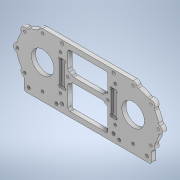
# Autodesk Inventor part: Trunk_lower_waisit_frame
Saved by Autodesk Inventor 2020.4 (Build 244396000, 396)
## iProperties
Created: 2021-09-21
Part Number: Trunk_lower_waisit_frame
Material: アルミニウム 2014-T4
Document SubType Name: Modeling
Designer: Masato Kubotera
Density: 2.8 g/cm^3
Appearance: 滑らか - 淡い灰色
Mass: 76.4309 g
Surface Area: 174.27 cm^2
Volume: 27.2967 cm^3
Description: A2017 T4
Author: Masato Kubotera
Autodesk Inventor part; units mm, degrees
ref_plane "YZ Plane" through (0, 0, 0) normal (1, 0, 0) x (0, 1, 0)
ref_plane "XZ Plane" through (0, 0, 0) normal (0, 1, 0) x (-1, 0, 0)
ref_plane "XY Plane" through (0, 0, 0) normal (0, 0, 1) x (1, 0, 0)
sketch "スケッチ1" plane through (0, 0, 0) normal (0, 0, 1) x (1, 0, 0)
  line L0 (-62, 30.75) -> (62, 30.75)
  line L1 (62, -30.75) -> (-62, -30.75)
  line L2 (-62, 30.75) -> (62, -30.75) construction
  line L3 (62, 30.75) -> (-62, -30.75) construction
  line L4 (0, 30.75) -> (0, -30.75) construction
  circle A0 centre (-44, 2.25) radius 10.5 construction
  line L5 (-57.5, 1.25) -> (-30.5, 1.25) construction
  line L6 (-30.5, 1.25) -> (-30.5, -25.75) construction
  line L7 (-30.5, -25.75) -> (-57.5, -25.75) construction
  line L8 (-57.5, -25.75) -> (-57.5, 1.25) construction
  line L9 (-44, 1.25) -> (-44, -25.75) construction
  line L10 (-57.5, -12.25) -> (-30.5, -12.25) construction
  circle A1 centre (-57.5, 1.25) radius 1.425 construction
  circle A2 centre (-57.5, -25.75) radius 1.425
  circle A3 centre (-30.5, 1.25) radius 1.425 construction
  circle A4 centre (-30.5, -25.75) radius 1.425
  line L11 (-27.5, 14.75) -> (-22.5, 14.75) construction
  line L12 (-22.5, 14.75) -> (-22.5, -10.25) construction
  line L13 (-22.5, -10.25) -> (-27.5, -10.25) construction
  line L14 (-27.5, -10.25) -> (-27.5, 14.75) construction
  line L15 (-27.5, 14.75) -> (-22.5, -10.25) construction
  line L16 (-22.5, 14.75) -> (-27.5, -10.25) construction
  line L17 (-27.51, 14.76) -> (-22.49, 14.76)
  line L18 (-22.49, 14.76) -> (-22.49, -10.26)
  line L19 (-22.49, -10.26) -> (-27.51, -10.26)
  line L20 (-27.51, -10.26) -> (-27.51, 14.76)
  line L21 (-27.51, 14.76) -> (-22.49, -10.26) construction
  line L22 (-22.49, 14.76) -> (-27.51, -10.26) construction
  line L23 (-27.51, 2.25) -> (-22.49, 2.25) construction
  line L24 (-25, 14.76) -> (-25, -10.26) construction
  arc A5 (-27.51, 14.76) -> (-27.51, 12.66) centre (-27.51, 13.71) ccw
  arc A6 (-22.49, 12.66) -> (-22.49, 14.76) centre (-22.49, 13.71) ccw
  arc A7 (-27.51, -8.16) -> (-27.51, -10.26) centre (-27.51, -9.21) ccw
  arc A8 (-22.49, -10.26) -> (-22.49, -8.16) centre (-22.49, -9.21) ccw
  circle A9 centre (-25, 27.75) radius 1.55
  line L25 (-22.5, -17.25) -> (-27.5, -17.25) construction
  circle A10 centre (-25, -23.25) radius 1.55
  circle A11 centre (-44, 2.25) radius 11
  line L26 (62, 2.25) -> (-62, 2.25) construction
  line L27 (-60, 14.25) -> (-28, 14.25) construction
  line L28 (-28, 14.25) -> (-28, -28.75) construction
  line L29 (-28, -28.75) -> (-60, -28.75) construction
  line L30 (-60, -28.75) -> (-60, 14.25) construction
  line L31 (-60, 14.25) -> (-28, -28.75) construction
  line L32 (-28, 14.25) -> (-60, -28.75) construction
  line L33 (-62, 30.75) -> (-62, -30.75) construction
  line L34 (62, 30.75) -> (62, -30.75) construction
  circle A12 centre (-44, 2.25) radius 12.5 construction
  circle A13 centre (-44, 2.25) radius 20.5 construction
  circle A14 centre (-44, 2.25) radius 28.5 construction
  circle A15 centre (-44, 26.75) radius 1.25
  circle A16 centre (-61.3241, 19.5741) radius 1.25
  circle A17 centre (-68.5, 2.25) radius 1.25
  circle A18 centre (-61.3241, -15.0741) radius 1.25
  circle A19 centre (-44, -22.25) radius 1.25
  circle A20 centre (-26.6759, -15.0741) radius 1.25
  circle A21 centre (-19.5, 2.25) radius 1.25
  circle A22 centre (-26.6759, 19.5741) radius 1.25
  line L35 (-62, -21.122) -> (-62, -30.75)
  circle A23 centre (57.5, 1.25) radius 1.425 construction
  circle A24 centre (57.5, -25.75) radius 1.425
  circle A25 centre (30.5, 1.25) radius 1.425 construction
  circle A26 centre (30.5, -25.75) radius 1.425
  line L36 (27.51, 14.76) -> (22.49, 14.76)
  line L37 (22.49, 14.76) -> (22.49, -10.26)
  line L38 (22.49, -10.26) -> (27.51, -10.26)
  line L39 (27.51, -10.26) -> (27.51, 14.76)
  arc A27 (27.51, 12.66) -> (27.51, 14.76) centre (27.51, 13.71) ccw
  arc A28 (22.49, 14.76) -> (22.49, 12.66) centre (22.49, 13.71) ccw
  arc A29 (22.49, -8.16) -> (22.49, -10.26) centre (22.49, -9.21) ccw
  arc A30 (27.51, -10.26) -> (27.51, -8.16) centre (27.51, -9.21) ccw
  circle A31 centre (25, 27.75) radius 1.55
  circle A32 centre (25, -23.25) radius 1.55
  circle A33 centre (44, 2.25) radius 11
  circle A34 centre (44, 26.75) radius 1.25
  circle A35 centre (61.3241, 19.5741) radius 1.25
  circle A36 centre (68.5, 2.25) radius 1.25
  circle A37 centre (61.3241, -15.0741) radius 1.25
  circle A38 centre (44, -22.25) radius 1.25
  circle A39 centre (26.6759, -15.0741) radius 1.25
  circle A40 centre (19.5, 2.25) radius 1.25
  circle A41 centre (26.6759, 19.5741) radius 1.25
  line L40 (62, -21.122) -> (62, -30.75)
  line L41 (-68.5, 2.25) -> (-73.5, 2.25) construction
  circle A42 centre (-26.6759, -15.0741) radius 6.25 construction
  circle A43 centre (-44, 2.25) radius 24.5 construction
  circle A44 centre (-30.5, -25.75) radius 2.4 construction
  arc A45 (-47.969, 27.2469) -> (-58.8689, 22.732) centre (-44, 2.25) ccw
  arc A46 (-44, 30.75) -> (-47.969, 27.2469) centre (-44, 26.75) ccw
  arc A47 (-58.8689, 22.732) -> (-64.482, 17.1189) centre (-61.3241, 19.5741) ccw
  arc A48 (-64.482, 17.1189) -> (-68.9969, 6.219) centre (-44, 2.25) ccw
  arc A49 (-68.9969, 6.219) -> (-68.9969, -1.719) centre (-68.5, 2.25) ccw
  arc A50 (-68.9969, -1.719) -> (-64.482, -12.6189) centre (-44, 2.25) ccw
  arc A51 (-64.482, -12.6189) -> (-62, -19.0166) centre (-61.3241, -15.0741) ccw
  line L42 (-62, -19.0166) -> (-62, -21.122)
  arc A52 (58.8689, 22.732) -> (47.969, 27.2469) centre (44, 2.25) ccw
  arc A53 (47.969, 27.2469) -> (44, 30.75) centre (44, 26.75) ccw
  arc A54 (64.482, 17.1189) -> (58.8689, 22.732) centre (61.3241, 19.5741) ccw
  arc A55 (68.9969, 6.219) -> (64.482, 17.1189) centre (44, 2.25) ccw
  arc A56 (68.9969, -1.719) -> (68.9969, 6.219) centre (68.5, 2.25) ccw
  arc A57 (64.482, -12.6189) -> (68.9969, -1.719) centre (44, 2.25) ccw
  arc A58 (62, -19.0166) -> (64.482, -12.6189) centre (61.3241, -15.0741) ccw
  line L43 (62, -19.0166) -> (62, -21.122)
  line L44 (19.5, 25.75) -> (-19.5, 25.75)
  line L45 (-19.5, 25.75) -> (-19.5, 7.25)
  circle A59 centre (-25, 27.75) radius 2.75 construction
  line L46 (-15.1699, 4.75) -> (15.1699, 4.75)
  arc A60 (-15.1699, 4.75) -> (-19.5, 7.25) centre (-19.5, 2.25) ccw
  line L47 (19.5, 25.75) -> (19.5, 7.25)
  arc A61 (19.5, 7.25) -> (15.1699, 4.75) centre (19.5, 2.25) ccw
  line L48 (-15.1699, -0.25) -> (15.1699, -0.25)
  arc A62 (-19.5, -2.75) -> (-15.1699, -0.25) centre (-19.5, 2.25) ccw
  arc A63 (15.1699, -0.25) -> (19.5, -2.75) centre (19.5, 2.25) ccw
  line L49 (-19.5, -2.75) -> (-19.5, -25.75)
  line L50 (-19.5, -25.75) -> (19.5, -25.75)
  line L51 (19.5, -25.75) -> (19.5, -2.75)
  point P0 (0, 0)
  point P1 (-25, 2.25)
  point P2 (-22.49, 12.66)
  point P3 (-22.49, -8.16)
  point P4 (-27.51, -8.16)
  point P5 (-44, -7.25)
  point P6 (22.49, -8.16)
  point P7 (22.49, 12.66)
  point P8 (27.9147, 19.7411)
  point P9 (27.51, 18.6431)
  point P10 (27.51, -8.16)
  point P11 (-27.51, 18.6431)
  point P12 (-27.9147, 19.7411)
  point P13 (-26.4271, 21.76)
  point P14 (-26.9247, 21.76)
  point P15 (-27.51, 20.5051)
  point P16 (27.51, 20.5051)
  point P17 (26.9247, 21.76)
  point P18 (26.4271, 21.76)
  point P19 (-47, 30.75)
  point P20 (47, 30.75)
  point P21 (-25, 2.25)
  dimension "d3" = 21
  dimension "d4" = 27
  dimension "d5" = 2.85
  dimension "d7" = 27
  dimension "d8" = 5
  dimension "d9" = 25
  dimension "d10" = 0.01
  dimension "d11" = 0.01
  dimension "d12" = 1.05
  dimension "d13" = 3.1
  dimension "d19" = 3.1
  dimension "d21" = 6
  dimension "d24" = 3
  dimension "d29" = 0.5
  dimension "d34" = 11.5
  dimension "d45" = 32
  dimension "d46" = 43
  dimension "d47" = 9.5
  dimension "d71" = 44
  dimension "d73" = 1
  dimension "d74" = 16.5
  dimension "d78" = 28.5
  dimension "d79" = 33
  dimension "d80" = 25
  dimension "d81" = 41
  dimension "d82" = 8
  dimension "d84" = 2.5
  dimension "d85" = 24.5
  dimension "d88" = 360
  dimension "d90" = 2
  dimension "d91" = 2
  dimension "d93" = 4
  dimension "d94" = 5
  dimension "d97" = 5
  dimension "d101" = 4.8
  dimension "d105" = 4
  dimension "d106" = 25.31
  dimension "d107" = 4
  dimension "d108" = 25.31
  dimension "d109" = 25.31
  dimension "d110" = 4
  dimension "d111" = 4
  dimension "d113" = 5.5
  dimension "d114" = 5
  dimension "d116" = 3
  dimension "d117" = 5
  dimension "d118" = 5
  dimension "d122" = 5
  dimension "d123" = 16
  dimension "d124" = 13
  constraints: 104 end point, 64 centre point, 61 symmetric about line, 54 point on circle, 19 coincident, 19 midpoint, 16 point on line, 10 parallel, 9 perpendicular, 8 horizontal, 4 vertical, 52 other
  measures "d3" diameter of A0
  measures "d4" distance of L6.end L7.end
  measures "d5" diameter of A1
  measures "d7" distance of L6.end L5.end
  measures "d8" distance of L12.end L13.end
  measures "d9" distance of L11.end L12.end
  measures "d10" distance between parallel lines of L17 L11
  measures "d11" distance between parallel lines of L18 L12
  measures "d12" radius of A5
  measures "d13" diameter of A9
  measures "d19" diameter of A10
  measures "d21" vertical distance of L25.start A10.centre
  measures "d24" vertical distance of L4.start A9.centre
  measures "d29" radial gap between concentric circles of A0 A11
  measures "d34" distance from line of A3.centre L13
  measures "d45" distance of L28.end L29.end
  measures "d46" distance of L27.end L28.end
  measures "d47" distance of point (-44, -7.25) A11.centre
  measures "d71" horizontal distance of point (0, 0) A0.centre
  measures "d73" distance of L9.start A11.centre
  measures "d74" horizontal distance of L11.start A0.centre
  measures "d78" distance from line of L26.end L0
  measures "d79" distance from line of L1 L26.end
  measures "d80" diameter of A12
  measures "d81" diameter of A13
  measures "d82" radial gap between concentric circles of A14 A13
  measures "d84" diameter of A15
  measures "d85" distance of A0.centre A15.centre
  measures "d90" horizontal distance of L1.end L29.end
  measures "d91" horizontal distance of L29.end L1.end
  measures "d93" distance from line of A15.centre L0
  measures "d94" distance of L41.start L41.end
  measures "d97" radial gap between concentric circles of A20 A42
  measures "d101" diameter of A44
  measures "d105" radius of A46
  measures "d106" radius of A45
  measures "d107" radius of A47
  measures "d108" radius of A48
  measures "d109" radius of A50
  measures "d110" radius of A49
  measures "d111" radius of A51
  measures "d113" diameter of A59
  measures "d114" distance from line of L44.end L0
  measures "d116" distance from line of L44.end L12
  measures "d117" distance between parallel lines of L48 L46
  measures "d118" distance between parallel lines of L1 L50
  measures "d122" radius of A60
  measures "d123" distance from line of L11.end L0
  measures "d124" distance from line of A10.centre L13
extrude "押し出し1" add sketch "スケッチ1" along normal blind 4
extrude "押し出し2" add sketch "スケッチ1" along normal blind 1.9 contours L17 L18 L19 L20 | L20 A5 | A6 L18 | L20 A7 | A8 L18 | L39 L38 L37 L36 | A27 L39 | L37 A28 | A30 L39 | L37 A29
fillet "フィレット1" radius 2 18 edges at (-62, -30.75, 2) (62, -30.75, 2) (64.482, -12.6189, 2) (62, -19.0166, 2) (68.9969, -1.719, 2) (64.482, 17.1189, 2) (68.9969, 6.219, 2) (58.8689, 22.732, 2) (47.969, 27.2469, 2) (44, 30.75, 2) (-44, 30.75, 2) (-47.969, 27.2469, 2) (-58.8689, 22.732, 2) (-64.482, 17.1189, 2) (-68.9969, 6.219, 2) (-68.9969, -1.719, 2) (-64.482, -12.6189, 2) (-62, -19.0166, 2)
fillet "フィレット2" radius 2 12 edges at (-19.5, 25.75, 2) (19.5, 25.75, 2) (15.1699, 4.75, 2) (-15.1699, 4.75, 2) (-19.5, -2.75, 2) (-15.1699, -0.25, 2) (15.1699, -0.25, 2) (19.5, -2.75, 2) (19.5, -25.75, 2) (-19.5, -25.75, 2) (-19.5, 7.25, 2) (19.5, 7.25, 2)
equation "\"d11\" = d10"
